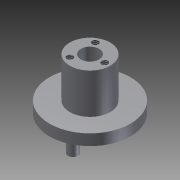
# Autodesk Inventor part: ss_inner_guide_bottom
Saved by Autodesk Inventor 2011 SP2 (Build 150309200, 309)
## iProperties
Created: 2012-05-25
Part Number: ss_inner_guide_bottom
Document SubType Name: Modeling
Designer: sungwook
Density: 1 g/cm^3
Author: sungwook
Autodesk Inventor part; units mm, degrees
ref_plane "YZ Plane" through (0, 0, 0) normal (1, 0, 0) x (0, 1, 0)
ref_plane "XZ Plane" through (0, 0, 0) normal (0, 1, 0) x (-1, 0, 0)
ref_plane "XY Plane" through (0, 0, 0) normal (0, 0, 1) x (1, 0, 0)
sketch "Sketch1" plane through (0, 0, 0) normal (0, 0, 1) x (1, 0, 0)
  circle A0 centre (0, 0) radius 5.5
  circle A1 centre (0, 0) radius 2.5
  dimension "d0" = 11
  dimension "d1" = 5
  constraints: 2 centre point, 2 coincident
  measures "d0" diameter of A0
  measures "d1" diameter of A1
extrude "Extrusion1" add sketch "Sketch1" along normal blind 13.923
sketch "Sketch2" plane through (0, 0, 0) normal (0, 0, -1) x (-1, 0, 0)
  circle A0 centre (0, 0) radius 5.5 projected
  circle A1 centre (0, 0) radius 11
  dimension "d4" = 22
  constraints: 1 centre point, 1 coincident
  measures "d4" diameter of A1
extrude "Extrusion2" add sketch "Sketch2" against normal blind 3
sketch "Sketch3" plane through (0, 0, 0) normal (0, 0, -1) x (-1, 0, 0)
  line L0 (-6.245, 5) -> (-3, 5)
  circle A0 centre (0, 0) radius 1.5
  line L1 (-3, 5) -> (-3, -5)
  line L2 (-3, -5) -> (-6.245, -5)
  circle A1 centre (9.494, -1.674) radius 0.85
  spline S0 degree 3 poles (10.2296, -1.2481) (10.2738, -1.3244) (10.307, -1.4092) (10.3385, -1.5597) (10.3447, -1.6214) (10.3436, -1.712) (10.3419, -1.74) (10.3365, -1.7883) (10.3335, -1.8088) (10.3258, -1.8503) (10.3211, -1.8713) (10.3072, -1.9234) (10.2972, -1.9541) (10.2556, -2.0601) (10.2157, -2.1299) (10.1087, -2.269) (10.0384, -2.3333) (9.8581, -2.452) (9.7422, -2.496) (9.5082, -2.5317) (9.39, -2.526) (9.1776, -2.4693) (9.0836, -2.4258) (8.9226, -2.3102) (8.8553, -2.243) (8.7497, -2.0936) (8.7103, -2.0147) (8.6611, -1.8594) (8.648, -1.7853) (8.6432, -1.6739) (8.644, -1.6375) (8.6494, -1.5744) (8.653, -1.5477) (8.6628, -1.4942) (8.669, -1.4673) (8.6873, -1.4034) (8.7006, -1.3666) (8.7492, -1.2563) (8.7927, -1.1869) (8.912, -1.0459) (8.9921, -0.9805) (9.1784, -0.8769) (9.2836, -0.8435) (9.5106, -0.8156) (9.6296, -0.8269) (9.8522, -0.8944) (9.955, -0.9506) (10.1164, -1.0872) (10.1799, -1.1623) (10.2296, -1.2481) knots -0.565469 -0.565469 -0.565469 -0.565469 -0.536596 -0.536596 -0.517611 -0.517611 -0.509175 -0.509175 -0.50297 -0.50297 -0.496493 -0.496493 -0.486731 -0.486731 -0.461904 -0.461904 -0.431221 -0.431221 -0.390112 -0.390112 -0.351113 -0.351113 -0.31806 -0.31806 -0.288721 -0.288721 -0.262067 -0.262067 -0.23952 -0.23952 -0.228596 -0.228596 -0.220512 -0.220512 -0.212256 -0.212256 -0.200543 -0.200543 -0.176006 -0.176006 -0.144684 -0.144684 -0.110272 -0.110272 -0.071492 -0.071492 -0.032498 -0.032498 0 0 0 0
  circle A2 centre (9.494, -1.674) radius 1.35
  arc A3 (0, -8) -> (-6.245, 5) centre (0, 0) ccw
  arc A4 (-6.245, -5) -> (0, -8) centre (0, 0) ccw
  circle A5 centre (-4.074, -8.737) radius 0.85
  spline S1 degree 3 poles (-3.2275, -8.6604) (-3.2176, -8.7695) (-3.229, -8.877) (-3.2876, -9.0751) (-3.3329, -9.1647) (-3.4588, -9.3344) (-3.5435, -9.4107) (-3.7198, -9.5152) (-3.8078, -9.5499) (-3.9747, -9.5845) (-4.0515, -9.5903) (-4.1887, -9.5813) (-4.248, -9.5712) (-4.333, -9.547) (-4.3592, -9.5382) (-4.4041, -9.5206) (-4.4229, -9.5123) (-4.4611, -9.4941) (-4.4802, -9.484) (-4.5275, -9.4567) (-4.5549, -9.4386) (-4.6492, -9.3685) (-4.7078, -9.3092) (-4.8155, -9.1642) (-4.8589, -9.0767) (-4.9231, -8.8674) (-4.9328, -8.7429) (-4.9006, -8.5082) (-4.8622, -8.3976) (-4.7491, -8.2109) (-4.6814, -8.1333) (-4.5263, -8.0114) (-4.4435, -7.9656) (-4.2507, -7.8985) (-4.1412, -7.8825) (-3.9721, -7.8911) (-3.9136, -7.9002) (-3.8251, -7.9236) (-3.7941, -7.9337) (-3.7394, -7.9552) (-3.7153, -7.9659) (-3.6658, -7.9908) (-3.6405, -8.0053) (-3.5776, -8.0455) (-3.5413, -8.0731) (-3.4268, -8.1755) (-3.361, -8.262) (-3.2655, -8.4537) (-3.2369, -8.5564) (-3.2275, -8.6604) knots -0.566086 -0.566086 -0.566086 -0.566086 -0.531825 -0.531825 -0.498779 -0.498779 -0.460694 -0.460694 -0.429612 -0.429612 -0.405256 -0.405256 -0.386838 -0.386838 -0.378505 -0.378505 -0.372312 -0.372312 -0.365791 -0.365791 -0.355852 -0.355852 -0.330056 -0.330056 -0.298514 -0.298514 -0.25701 -0.25701 -0.218398 -0.218398 -0.185587 -0.185587 -0.156394 -0.156394 -0.123104 -0.123104 -0.105349 -0.105349 -0.095573 -0.095573 -0.087672 -0.087672 -0.078924 -0.078924 -0.065227 -0.065227 -0.032657 -0.032657 0 0 0 0
  circle A6 centre (-4.074, -8.737) radius 1.35
  circle A7 centre (-4.82, 8.349) radius 0.85
  spline S2 degree 3 poles (-4.1123, 8.8197) (-4.052, 8.7291) (-4.0084, 8.6259) (-3.9677, 8.4209) (-3.9647, 8.3234) (-3.9919, 8.1375) (-4.0188, 8.0509) (-4.0994, 7.8893) (-4.1522, 7.8154) (-4.2455, 7.7212) (-4.2773, 7.6934) (-4.3337, 7.6513) (-4.3572, 7.6355) (-4.4041, 7.6072) (-4.4275, 7.5946) (-4.4822, 7.5683) (-4.5139, 7.5553) (-4.6086, 7.5231) (-4.6731, 7.5092) (-4.8426, 7.4929) (-4.947, 7.5022) (-5.1521, 7.5589) (-5.2492, 7.6077) (-5.4281, 7.7434) (-5.5042, 7.8321) (-5.6193, 8.0357) (-5.6549, 8.1509) (-5.6758, 8.3693) (-5.6674, 8.4725) (-5.6185, 8.6517) (-5.5851, 8.7291) (-5.4963, 8.8702) (-5.4427, 8.9337) (-5.3552, 9.0101) (-5.3302, 9.0296) (-5.2865, 9.0599) (-5.2685, 9.0714) (-5.2323, 9.0926) (-5.2143, 9.1023) (-5.1705, 9.1239) (-5.1446, 9.1351) (-5.0727, 9.162) (-5.0263, 9.175) (-4.8823, 9.2025) (-4.7852, 9.2034) (-4.5796, 9.1723) (-4.4735, 9.1329) (-4.2735, 9.0117) (-4.182, 8.9246) (-4.1123, 8.8197) knots -0.567177 -0.567177 -0.567177 -0.567177 -0.53086 -0.53086 -0.500336 -0.500336 -0.472721 -0.472721 -0.445441 -0.445441 -0.432747 -0.432747 -0.42424 -0.42424 -0.416254 -0.416254 -0.405955 -0.405955 -0.386117 -0.386117 -0.354442 -0.354442 -0.320748 -0.320748 -0.283148 -0.283148 -0.243084 -0.243084 -0.208567 -0.208567 -0.181377 -0.181377 -0.155642 -0.155642 -0.146036 -0.146036 -0.139581 -0.139581 -0.133402 -0.133402 -0.124853 -0.124853 -0.110096 -0.110096 -0.079394 -0.079394 -0.04201 -0.04201 0 0 0 0
  circle A8 centre (-4.82, 8.349) radius 1.35
  circle A9 centre (0, 0) radius 1.5
  circle A10 centre (0, 0) radius 8
  dimension "d7" = 2.7
  dimension "d8" = 2.7
  dimension "d9" = 2.7
  constraints: 7 centre point, 6 end point, 4 point on circle, 1 coincident, 1 vertical alignment, 12 other
  measures "d7" diameter of A2
  measures "d8" diameter of A6
  measures "d9" diameter of A8
extrude "Extrusion3" add sketch "Sketch3" along normal blind 3 contours A1 | A2 | A5 | A6 | A7 | A8
sketch "Sketch4" plane through (0, 0, 13.923) normal (0, 0, 1) x (1, 0, 0)
  circle A0 centre (0, 0) radius 2.5 projected
  line L0 (-7.7, 0) -> (7.7, 0) projected
  point P0 (4, 0)
  dimension "d12" = 4
  constraints: 1 point on line
  measures "d12" distance of point (4, 0) A0.centre
hole "Hole1" at (4, 0, 13.923) direction (0, 0, -1) diameter 1.694 depth 3 thread size "2-56 UNC" class "2B" standard "ANSI Unified Screw Threads"
pattern_circular "Circular Pattern1" count 3 over 360 about axis through (0, 0, -10) along (0, 0, 1) of "Hole1"
sketch "Sketch5" plane through (4.074, -8.737, -3) normal (0, 0, -1) x (-1, 0, 0)
  circle A0 centre (0, 0) radius 1.35 projected
  point P0 (4.074, 8.737)
hole "Hole2" at (4.074, -8.737, -3) direction (0, 0, 1) diameter 1.694 depth 3 tip angle 118 thread size "2-56 UNC" class "2B" standard "ANSI Unified Screw Threads"
body "Solid1"
